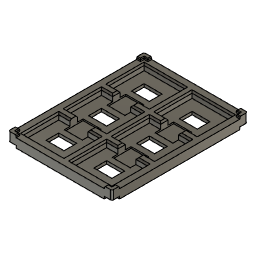
CPU_Tray_LGA_2011-0 (Autodesk Fusion 360 design; units mm, degrees)
Autodesk Fusion 360 part; units mm, degrees
sketch "Esquisse1" plane through (0, 0, 0) normal (0, 0, 1) x (1, 0, 0)
  line L0 (0, 0) -> (69, 0)
  line L1 (69, -181) -> (0, -181)
  line L2 (0, -181) -> (0, 0)
  line L3 (10, -10) -> (64, -10)
  line L4 (64, -10) -> (64, -57)
  line L5 (64, -57) -> (10, -57)
  line L6 (10, -57) -> (10, -10)
  line L7 (25, -25) -> (49, -25)
  line L8 (49, -25) -> (49, -42)
  line L9 (49, -42) -> (25, -42)
  line L10 (25, -42) -> (25, -25)
  line L11 (49, -99) -> (25, -99)
  line L12 (64, -114) -> (10, -114)
  line L13 (10, -114) -> (10, -67)
  line L14 (49, -82) -> (49, -99)
  line L15 (25, -99) -> (25, -82)
  line L16 (10, -67) -> (64, -67)
  line L17 (25, -82) -> (49, -82)
  line L18 (64, -67) -> (64, -114)
  line L19 (64, -171) -> (10, -171)
  line L20 (64, -124) -> (64, -171)
  line L21 (49, -156) -> (25, -156)
  line L22 (10, -171) -> (10, -124)
  line L23 (25, -139) -> (49, -139)
  line L24 (25, -156) -> (25, -139)
  line L25 (49, -139) -> (49, -156)
  line L26 (10, -124) -> (64, -124)
  line L27 (74, -67) -> (74, -114)
  line L28 (113, -139) -> (89, -139)
  line L29 (89, -99) -> (113, -99)
  line L30 (74, -171) -> (128, -171)
  line L31 (113, -156) -> (113, -139)
  line L32 (128, -57) -> (128, -10)
  line L33 (113, -25) -> (89, -25)
  line L34 (138, -181) -> (138, 0)
  line L35 (74, -124) -> (74, -171)
  line L36 (113, -82) -> (89, -82)
  line L37 (128, -124) -> (74, -124)
  line L38 (128, -114) -> (128, -67)
  line L39 (74, -57) -> (128, -57)
  line L40 (128, -171) -> (128, -124)
  line L41 (128, -10) -> (74, -10)
  line L42 (89, -156) -> (113, -156)
  line L43 (74, -114) -> (128, -114)
  line L44 (89, -42) -> (113, -42)
  line L45 (89, -139) -> (89, -156)
  line L46 (128, -67) -> (74, -67)
  line L47 (113, -99) -> (113, -82)
  line L48 (89, -25) -> (89, -42)
  line L49 (74, -10) -> (74, -57)
  line L50 (89, -82) -> (89, -99)
  line L51 (113, -42) -> (113, -25)
  line L52 (138, 0) -> (69, 0)
  line L53 (69, -181) -> (138, -181)
  point P0 (138, 0)
  dimension "d3" = 47
  dimension "d4" = 54
  dimension "d7" = 15
  dimension "d8" = 15
  dimension "d9" = 15
  dimension "d10" = 15
  dimension "d11" = 10
  dimension "d13" = 47
  dimension "d14" = 54
  dimension "d15" = 15
  dimension "d16" = 15
  dimension "d17" = 15
  dimension "d18" = 15
  dimension "d19" = 47
  dimension "d20" = 54
  dimension "d21" = 15
  dimension "d22" = 15
  dimension "d23" = 15
  dimension "d24" = 15
  dimension "d25" = 10
  dimension "d26" = 10
  dimension "d27" = 10
  dimension "d28" = 10
  constraint horizontal L0
  constraint horizontal L1
  constraint vertical L2
  constraint coincident L0.start L2.end
  constraint horizontal L3
  constraint vertical L4
  constraint horizontal L5
  constraint vertical L6
  constraint horizontal L7
  constraint vertical L8
  constraint horizontal L9
  constraint vertical L10
  constraint horizontal L16
  constraint vertical L18
  constraint horizontal L12
  constraint vertical L13
  constraint horizontal L17
  constraint vertical L14
  constraint horizontal L11
  constraint vertical L15
  constraint horizontal L26
  constraint vertical L20
  constraint horizontal L19
  constraint vertical L22
  constraint horizontal L23
  constraint vertical L25
  constraint horizontal L21
  constraint vertical L24
  measures "d3" distance of L3 L5
  measures "d4" distance of L4 L6
  measures "d7" distance of L6 L10
  measures "d8" distance of L5 L9
  measures "d9" distance of L4 L8
  measures "d10" distance of L3 L7
  measures "d11" distance of L2 L6
  measures "d13" distance of L12 L16
  measures "d14" distance of L13 L18
  measures "d15" distance of L13 L15
  measures "d16" distance of L11 L12
  measures "d17" distance of L14 L18
  measures "d18" distance of L16 L17
  measures "d19" distance of L19 L26
  measures "d20" distance of L20 L22
  measures "d21" distance of L22 L24
  measures "d22" distance of L19 L21
  measures "d23" distance of L20 L25
  measures "d24" distance of L23 L26
  measures "d25" distance of L5 L16
  measures "d26" distance of L12 L26
  measures "d27" distance of L0 L3
  measures "d28" distance of L1 L19
extrude "Extrusion1" add sketch "Esquisse1" along normal blind 4 contours L3 L4 L5 L6 | L12 L13 L16 L18 | L19 L20 L22 L26 | L27 L38 L43 L46 | L30 L35 L37 L40 | L32 L39 L41 L49 makes body 1 at (33, -109, 0) makes body 2 at (41, -52, 0) makes body 3 at (33, -166, 0) makes body 4 at (105, -109, 0) makes body 5 at (97, -52, 0) makes body 6 at (97, -166, 0)
extrude "Extrusion2" add sketch "Esquisse1" along normal blind 12 contours L0 L1 L2 L34 L52 L53 bodies 1 2 3 4 5 6
sketch "Esquisse2" plane through (0, 0, 12) normal (0, 0, 1) x (-1, 0, 0)
  line L0 (-10, 67) -> (-64, 67)
  line L1 (-64, 67) -> (-64, 114)
  line L2 (-64, 114) -> (-10, 114)
  line L3 (-10, 114) -> (-10, 67)
  line L4 (-10, 171) -> (-10, 124)
  line L5 (-10, 124) -> (-64, 124)
  line L6 (-64, 124) -> (-64, 171)
  line L7 (-64, 171) -> (-10, 171)
  line L8 (-74, 57) -> (-74, 10)
  line L9 (-74, 10) -> (-128, 10)
  line L10 (-128, 10) -> (-128, 57)
  line L11 (-128, 57) -> (-74, 57)
  line L12 (-128, 124) -> (-128, 171)
  line L13 (-128, 171) -> (-74, 171)
  line L14 (-74, 171) -> (-74, 124)
  line L15 (-74, 124) -> (-128, 124)
  line L16 (-74, 67) -> (-128, 67)
  line L17 (-128, 67) -> (-128, 114)
  line L18 (-128, 114) -> (-74, 114)
  line L19 (-74, 114) -> (-74, 67)
  line L20 (-64, 57) -> (-10, 57)
  line L21 (-10, 57) -> (-10, 10)
  line L22 (-10, 10) -> (-64, 10)
  line L23 (-64, 10) -> (-64, 57)
  line L24 (0, 181) -> (-138, 181)
  line L25 (-138, 181) -> (-138, 0)
  line L26 (-138, 0) -> (0, 0)
  line L27 (-25, 49.5) -> (-49, 49.5)
  line L28 (-49, 49.5) -> (-49, 74.5)
  line L29 (-49, 74.5) -> (-25, 74.5)
  line L30 (-25, 74.5) -> (-25, 49.5)
  line L31 (-25, 42) -> (-25, 25)
  line L32 (-49, 25) -> (-49, 42)
  line L33 (-25, 106.5) -> (-49, 106.5)
  line L34 (-49, 106.5) -> (-49, 131.5)
  line L35 (-49, 131.5) -> (-25, 131.5)
  line L36 (-25, 131.5) -> (-25, 106.5)
  line L37 (-25, 99) -> (-25, 82)
  line L38 (-49, 82) -> (-49, 99)
  line L39 (-69, 0) -> (-69, 181)
  line L40 (-113, 131.5) -> (-113, 106.5)
  line L41 (-89, 106.5) -> (-89, 131.5)
  line L42 (-113, 106.5) -> (-89, 106.5)
  line L43 (-89, 131.5) -> (-113, 131.5)
  line L44 (-113, 74.5) -> (-113, 49.5)
  line L45 (-89, 82) -> (-89, 99)
  line L46 (-89, 49.5) -> (-89, 74.5)
  line L47 (-113, 99) -> (-113, 82)
  line L48 (-89, 25) -> (-89, 42)
  line L49 (-113, 42) -> (-113, 25)
  line L50 (-113, 49.5) -> (-89, 49.5)
  line L51 (-89, 74.5) -> (-113, 74.5)
  dimension "d34" = 25
  dimension "d41" = 25
  dimension "d43" = 7.5
  dimension "d44" = 10
  dimension "d45" = 7.5
  constraint horizontal L27
  constraint vertical L28
  constraint horizontal L29
  constraint vertical L30
  constraint collinear L30 L31
  constraint collinear L28 L32
  constraint horizontal L33
  constraint vertical L34
  constraint horizontal L35
  constraint vertical L36
  constraint collinear L36 L37
  constraint collinear L34 L38
  constraint midpoint L26 L39.start
  constraint midpoint L24 L39.end
  constraint symmetric L27.start L39 L44.end
  constraint symmetric L27.end L39 L46.start
  constraint symmetric L28.end L39 L46.end
  constraint symmetric L29.end L39 L44.start
  constraint symmetric L31.start L39 L49.start
  constraint symmetric L31.end L39 L49.end
  constraint symmetric L32.start L39 L48.start
  constraint symmetric L32.end L39 L48.end
  constraint symmetric L33.start L39 L40.end
  constraint symmetric L33.end L39 L41.start
  constraint symmetric L34.end L39 L41.end
  constraint symmetric L35.end L39 L40.start
  constraint symmetric L37.start L39 L47.start
  constraint symmetric L37.end L39 L47.end
  constraint symmetric L38.start L39 L45.start
  constraint symmetric L38.end L39 L45.end
  measures "d34" distance of L27 L29
  measures "d41" distance of L33 L35
  measures "d43" distance of L20 L27
  measures "d44" distance of L0 L20
  measures "d45" distance of L2 L33
extrude "Extrusion3" cut sketch "Esquisse2" against normal blind 10 contours L0 L20 L28 L30 | L0 L28 L29 L30 | L20 L27 L28 L30 | L2 L33 L34 L36 | L2 L5 L34 L36 | L5 L34 L35 L36 | L11 L44 L46 L50 | L11 L16 L44 L46 | L16 L44 L46 L51 | L18 L40 L41 L42 | L15 L18 L40 L41 | L15 L40 L41 L43 bodies 1
sketch "Esquisse3" plane through (0, 0, 12) normal (0, 0, 1) x (-1, 0, 0)
  line L0 (0, 181) -> (-138, 181)
  line L1 (-138, 181) -> (-138, 0)
  line L2 (-138, 0) -> (0, 0)
  line L3 (0, 0) -> (0, 181)
  line L4 (-113, 57) -> (-113, 67)
  line L5 (-113, 67) -> (-128, 67)
  line L6 (-128, 67) -> (-128, 114)
  line L7 (-128, 114) -> (-113, 114)
  line L8 (-113, 114) -> (-113, 124)
  line L9 (-113, 124) -> (-128, 124)
  line L10 (-128, 124) -> (-128, 171)
  line L11 (-128, 171) -> (-74, 171)
  line L12 (-74, 171) -> (-74, 124)
  line L13 (-74, 124) -> (-89, 124)
  line L14 (-89, 124) -> (-89, 114)
  line L15 (-89, 114) -> (-74, 114)
  line L16 (-74, 114) -> (-74, 67)
  line L17 (-74, 67) -> (-89, 67)
  line L18 (-89, 67) -> (-89, 57)
  line L19 (-89, 57) -> (-74, 57)
  line L20 (-74, 57) -> (-74, 10)
  line L21 (-74, 10) -> (-128, 10)
  line L22 (-128, 10) -> (-128, 57)
  line L23 (-128, 57) -> (-113, 57)
  line L24 (-49, 57) -> (-49, 67)
  line L25 (-49, 67) -> (-64, 67)
  line L26 (-64, 67) -> (-64, 114)
  line L27 (-64, 114) -> (-49, 114)
  line L28 (-49, 114) -> (-49, 124)
  line L29 (-49, 124) -> (-64, 124)
  line L30 (-64, 124) -> (-64, 171)
  line L31 (-64, 171) -> (-10, 171)
  line L32 (-10, 171) -> (-10, 124)
  line L33 (-10, 124) -> (-25, 124)
  line L34 (-25, 124) -> (-25, 114)
  line L35 (-25, 114) -> (-10, 114)
  line L36 (-10, 114) -> (-10, 67)
  line L37 (-10, 67) -> (-25, 67)
  line L38 (-25, 67) -> (-25, 57)
  line L39 (-25, 57) -> (-10, 57)
  line L40 (-10, 57) -> (-10, 10)
  line L41 (-10, 10) -> (-64, 10)
  line L42 (-64, 10) -> (-64, 57)
  line L43 (-64, 57) -> (-49, 57)
  line L44 (0, 0) -> (0, 10)
  line L45 (-5, 10) -> (-5, 5)
  line L46 (-5, 5) -> (-10, 5)
  line L47 (-10, 5) -> (-10, 0)
  line L48 (0, 0) -> (-10, 0)
  line L49 (-5, 10) -> (0, 10)
  line L50 (-69, 0) -> (-69, 181)
  line L51 (0, 90.5) -> (-138, 90.5)
  line L52 (-133, 5) -> (-128, 5)
  line L53 (-138, 0) -> (-138, 10)
  line L54 (-133, 10) -> (-138, 10)
  line L55 (-138, 0) -> (-128, 0)
  line L56 (-133, 10) -> (-133, 5)
  line L57 (-128, 5) -> (-128, 0)
  line L58 (-133, 176) -> (-128, 176)
  line L59 (-5, 176) -> (-10, 176)
  line L60 (-5, 171) -> (0, 171)
  line L61 (0, 181) -> (-10, 181)
  line L62 (-133, 171) -> (-138, 171)
  line L63 (-128, 176) -> (-128, 181)
  line L64 (-133, 171) -> (-133, 176)
  line L65 (-10, 176) -> (-10, 181)
  line L66 (-138, 181) -> (-128, 181)
  line L67 (-138, 181) -> (-138, 171)
  line L68 (0, 181) -> (0, 171)
  line L69 (-5, 171) -> (-5, 176)
  point P0 (-138, 0)
  point P1 (-138, 0)
  point P2 (-138, 181)
  point P3 (-138, 181)
  point P4 (-74, 171)
  point P5 (0, 181)
  point P6 (-128, 171)
  point P7 (-64, 171)
  point P8 (0, 181)
  point P9 (-138, 181)
  point P10 (-10, 171)
  point P11 (-69, 181)
  constraint coincident L2.end L3.start
  constraint coincident L3 L44.end
  constraint perpendicular L2 L44
  constraint perpendicular L2 L45
  constraint perpendicular L45 L46
  constraint coincident L2 L47.end
  constraint perpendicular L2 L47
  constraint perpendicular L44 L49
  constraint midpoint L2 L50.start
  constraint midpoint L0 P11
  constraint midpoint L3 L51.start
  constraint midpoint L1 L51.end
  constraint symmetric L2.end L50 P1
  constraint symmetric L44.end L50 L53.end
  constraint symmetric L45.start L50 L54.start
  constraint symmetric L45.end L50 L52.start
  constraint symmetric L46.end L50 L52.end
  constraint symmetric L47.end L50 L55.end
  constraint symmetric L2.end L51 P8
  constraint symmetric P1 L51 P9
  constraint symmetric L20.end L51 P4
  constraint symmetric L21.end L51 P6
  constraint symmetric L40.end L51 P10
  constraint symmetric L41.end L51 P7
  constraint symmetric L44.end L51 L60.end
  constraint symmetric L45.start L51 L60.start
  constraint symmetric L45.end L51 L59.start
  constraint symmetric L46.end L51 L59.end
  constraint symmetric L47.end L51 L61.end
  constraint symmetric L50.start L51 P11
  constraint symmetric L51 P1 P9
  constraint symmetric L51 L53.end L62.end
  constraint symmetric L51 L55.end L63.end
  constraint symmetric L51 L52.start L58.start
  constraint symmetric L51 L54.start L62.start
  constraint symmetric L51 L52.end L58.end
extrude "Extrusion4" add sketch "Esquisse3" along normal blind 3 contours L0 L3 L59 L60 L61 L65 L68 L69 | L0 L1 L58 L62 L63 L64 L66 L67 | L2 L3 L44 L45 L46 L47 L48 L49 | L1 L2 L52 L53 L54 L55 L56 L57 bodies 1
sketch "Esquisse4" plane through (0, 0, 0) normal (0, 0, -1) x (1, 0, 0)
  line L0 (49, 139) -> (25, 139)
  line L1 (25, 139) -> (25, 156)
  line L2 (25, 156) -> (49, 156)
  line L3 (49, 156) -> (49, 139)
  line L4 (25, 42) -> (49, 42)
  line L5 (49, 42) -> (49, 25)
  line L6 (49, 25) -> (25, 25)
  line L7 (25, 25) -> (25, 42)
  line L8 (89, 139) -> (89, 156)
  line L9 (89, 156) -> (113, 156)
  line L10 (113, 156) -> (113, 139)
  line L11 (113, 139) -> (89, 139)
  line L12 (138, 181) -> (0, 181)
  line L13 (0, 181) -> (0, 0)
  line L14 (0, 0) -> (138, 0)
  line L15 (138, 0) -> (138, 181)
  line L16 (89, 82) -> (89, 99)
  line L17 (89, 99) -> (113, 99)
  line L18 (113, 99) -> (113, 82)
  line L19 (113, 82) -> (89, 82)
  line L20 (25, 82) -> (25, 99)
  line L21 (25, 99) -> (49, 99)
  line L22 (49, 99) -> (49, 82)
  line L23 (49, 82) -> (25, 82)
  line L24 (113, 42) -> (113, 25)
  line L25 (113, 25) -> (89, 25)
  line L26 (89, 25) -> (89, 42)
  line L27 (89, 42) -> (113, 42)
  line L28 (0, 0) -> (0, 10.2)
  line L29 (5.1, 10.2) -> (5.1, 5.1)
  line L30 (5.1, 5.1) -> (10.2, 5.1)
  line L31 (10.2, 5.1) -> (10.2, 0)
  line L32 (0, 10.2) -> (5.1, 10.2)
  line L33 (69, 181) -> (69, 0)
  line L34 (0, 90.5) -> (138, 90.5)
  line L35 (138, 0) -> (138, 10.2)
  line L36 (138, 10.2) -> (132.9, 10.2)
  line L37 (132.9, 10.2) -> (132.9, 5.1)
  line L38 (132.9, 5.1) -> (127.8, 5.1)
  line L39 (127.8, 5.1) -> (127.8, 0)
  line L40 (0, 0) -> (10.2, 0)
  line L41 (127.8, 0) -> (138, 0)
  line L42 (0, 170.8) -> (5.1, 170.8)
  line L43 (5.1, 170.8) -> (5.1, 175.9)
  line L44 (5.1, 175.9) -> (10.2, 175.9)
  line L45 (10.2, 175.9) -> (10.2, 181)
  line L46 (0, 181) -> (10.2, 181)
  line L47 (132.9, 175.9) -> (127.8, 175.9)
  line L48 (127.8, 175.9) -> (127.8, 181)
  line L49 (127.8, 181) -> (138, 181)
  line L50 (138, 181) -> (138, 170.8)
  line L51 (138, 170.8) -> (132.9, 170.8)
  line L52 (132.9, 170.8) -> (132.9, 175.9)
  line L53 (0, 181) -> (0, 170.8)
  dimension "d52" = 5.1
  dimension "d53" = 5.1
  dimension "d54" = 5.1
  dimension "d55" = 10.2
  dimension "d56" = 10.2
  dimension "d57" = 5.1
  constraint coincident L13.end L14.start
  constraint coincident L13 L28.end
  constraint perpendicular L14 L28
  constraint perpendicular L14 L29
  constraint perpendicular L29 L30
  constraint coincident L14 L31.end
  constraint perpendicular L14 L31
  constraint perpendicular L29 L32
  constraint midpoint L12 L33.start
  constraint midpoint L14 L33.end
  constraint midpoint L13 L34.start
  constraint midpoint L15 L34.end
  constraint symmetric L13.end L33 L14.end
  constraint symmetric L28.end L33 L35.end
  constraint symmetric L29.start L33 L36.end
  constraint symmetric L29.end L33 L37.end
  constraint symmetric L30.end L33 L38.end
  constraint symmetric L31.end L33 L39.end
  constraint symmetric L13.end L34 L12.end
  constraint symmetric L28.end L34 L42.start
  constraint symmetric L29.start L34 L42.end
  constraint symmetric L29.end L34 L43.end
  constraint symmetric L30.end L34 L44.end
  constraint symmetric L31.end L34 L45.end
  constraint symmetric L34 L14.end L12.start
  constraint symmetric L34 L35.end L50.end
  constraint symmetric L34 L36.end L51.end
  constraint symmetric L34 L37.end L47.start
  constraint symmetric L34 L38.end L47.end
  constraint symmetric L34 L39.end L48.end
  constraint symmetric L34 L13.end L12.end
  measures "d52" distance of L28 L29
  measures "d53" distance of L29.start L29.end
  measures "d54" distance of L29.end L30.end
  measures "d55" distance of L14 L32
  measures "d56" distance of L28 L31
  measures "d57" distance of L30.end L31.end
extrude "Extrusion5" cut sketch "Esquisse4" against normal blind 3.1 contours L12 L15 L47 L48 L49 L50 L51 L52 | L12 L13 L42 L43 L44 L45 L46 L53 | L14 L15 L35 L36 L37 L38 L39 L41 | L13 L14 L28 L29 L30 L31 L32 L40 bodies 1
chamfer "Chanfrein1" distance 2 angle 45 39 edges at (10, -33.5, 12) (37, -10, 12) (64, -33.5, 12) (74, -33.5, 12) (101, -10, 12) (128, -33.5, 12) (120.5, -57, 12) (81.5, -67, 12) (89, -62, 12) (81.5, -57, 12) (113, -62, 12) (120.5, -67, 12) (128, -90.5, 12) (120.5, -114, 12) (113, -119, 12) (120.5, -124, 12) (128, -147.5, 12) (101, -171, 12) (74, -147.5, 12) (81.5, -124, 12) (89, -119, 12) (81.5, -114, 12) (74, -90.5, 12) (49, -62, 12) (56.5, -67, 12) (56.5, -57, 12) (64, -90.5, 12) (56.5, -114, 12) (49, -119, 12) (56.5, -124, 12) (64, -147.5, 12) (37, -171, 12) (10, -147.5, 12) (17.5, -124, 12) (17.5, -114, 12) (10, -90.5, 12) (17.5, -67, 12) (25, -62, 12) (17.5, -57, 12) on bodies 1
chamfer "Chanfrein2" distance 1 angle 45 16 edges at (2.5, -171, 15) (5, -173.5, 15) (7.5, -176, 15) (10, -178.5, 15) (128, -178.5, 15) (130.5, -176, 15) (133, -173.5, 15) (135.5, -171, 15) (130.5, -5, 15) (128, -2.5, 15) (135.5, -10, 15) (133, -7.5, 15) (2.5, -10, 15) (5, -7.5, 15) (7.5, -5, 15) (10, -2.5, 15) on bodies 1
fillet "Congé1" radius 2 4 edges at (138, -181, 9.05) (0, -181, 9.05) (138, 0, 9.05) (0, 0, 9.05) on bodies 1
equation "d37 = 47.00 mm"
equation "d38 = ( d39 + d37 ) - ( d34 / 4 )"
equation "d39 = 10.00 mm"
equation "d41 = d34"
equation "d43 = ( d34 - d44 ) / 2"
equation "d45 = d43"
